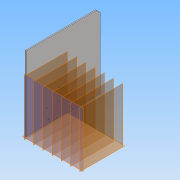
# Autodesk Inventor part: Selection_LHS
Saved by Autodesk Inventor 2018.1 (Build 221171000, 171)
## iProperties
Created: 2019-02-07
Part Number: Selection_LHS
Material: Generic
Document SubType Name: Modeling
Designer: James
Density: 1 g/cm^3
Appearance: Default
Author: James
Autodesk Inventor part; units mm, degrees
ref_plane "YZ Plane" through (0, 0, 0) normal (1, 0, 0) x (0, 1, 0)
ref_plane "XZ Plane" through (0, 0, 0) normal (0, 1, 0) x (-1, 0, 0)
ref_plane "XY Plane" through (0, 0, 0) normal (0, 0, 1) x (1, 0, 0)
derived "Selection_Skeleton.ipt"
ref_plane "Ground" through (0, 0, 0) normal (0, 1, 0) x (-1, 0, 0)
ref_plane "LHS inner" through (0, 0, 0) normal (1, 0, 0) x (0, 1, 0)
ref_plane "RHS inner" through (300, 0, 0) normal (1, 0, 0) x (0, 1, 0)
ref_plane "Lane 1" through (50, 0, 0) normal (1, 0, 0) x (0, 1, 0)
ref_plane "Lane 2" through (100, 0, 0) normal (1, 0, 0) x (0, 1, 0)
ref_plane "Lane 3" through (150, 0, 0) normal (1, 0, 0) x (0, 1, 0)
ref_plane "Lane 4" through (200, 0, 0) normal (1, 0, 0) x (0, 1, 0)
ref_plane "Lane 5" through (250, 0, 0) normal (1, 0, 0) x (0, 1, 0)
ref_plane "Back" through (0, 0, 0) normal (0, 0, 1) x (1, 0, 0)
sketch "Sketch1" plane through (0, 0, 0) normal (1, 0, 0) x (0, 1, 0)
  line L0 (-80, 0) -> (480, 0) projected
  line L1 (0, 480) -> (0, -80) projected
  line L2 (0, 0) -> (400, 0)
  line L3 (400, 0) -> (400, 400)
  line L4 (400, 400) -> (0, 400)
  line L5 (0, 400) -> (0, 0)
  dimension "d1" = 400
  dimension "d2" = 400
  constraints: 8 end point, 2 parallel, 1 horizontal, 1 perpendicular
  measures "d1" distance of L2.start L2.end
  measures "d2" distance of L2.end L3.end
extrude "Extrusion1" add sketch "Sketch1" against normal blind 5
chamfer "Chamfer1" distance 20 angle 45 1 edges at (-2.5, 400, 400)
sketch "Sketch2" plane through (-5, 0, 0) normal (-1, 0, 0) x (0, 0, 1)
  line L0 (0, 400) -> (0, 0) projected
  line L1 (0, 0) -> (400, 0) projected
  point P0 (20, 240)
  point P1 (79.1608, 230)
  point P2 (139.1608, 180)
  point P3 (80, 170)
  point P4 (20, 120)
  point P5 (79.1608, 110)
  dimension "d8" = 20
  dimension "d11" = 60
  dimension "d12" = 10
  dimension "d13" = 10
  dimension "d14" = 10
  dimension "d15" = 50
  dimension "d16" = 50
  dimension "d17" = 110
  dimension "d25" = 60
  dimension "d26" = 60
  constraints: 2 vertical alignment
  measures "d8" distance from line of point (20, 240) L0
  measures "d11" horizontal distance of point (139.161, 180) point (79.161, 230)
  measures "d12" vertical distance of point (79.161, 230) point (20, 240)
  measures "d13" vertical distance of point (139.161, 180) point (80, 170)
  measures "d14" vertical distance of point (79.161, 110) point (20, 120)
  measures "d15" vertical distance of point (139.161, 180) point (79.161, 230)
  measures "d16" vertical distance of point (80, 170) point (20, 120)
  measures "d17" distance from line of point (79.161, 110) L1
  measures "d25" distance of point (79.161, 230) point (20, 240)
  measures "d26" distance of point (139.161, 180) point (80, 170)
hole "Hole1" at (-5, 240, 20) at (-5, 230, 79.1608) at (-5, 180, 139.1608) at (-5, 170, 80) at (-5, 120, 20) at (-5, 110, 79.1608) direction (1, 0, 0) diameter 4.5 end through all clearance for "Socket Head Cap Screw" size "M4" standard "Ansi Metric M Profile"
equation "\"d13\" = d12"
equation "\"d14\" = d13"
equation "\"d16\" = d15"
equation "\"d26\" = d25"
body "Solid1"
